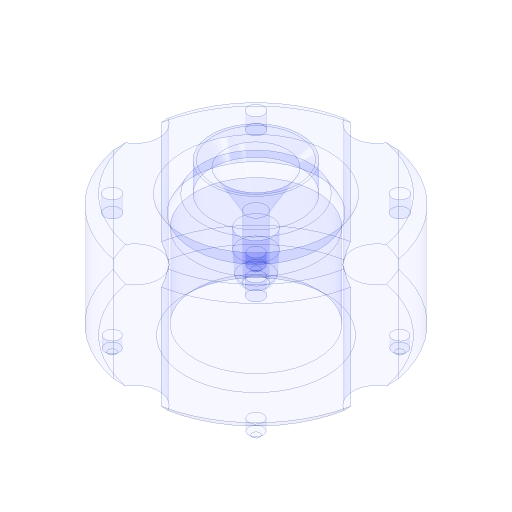
# Autodesk Inventor part: cpd_lowrcf_1.3_p3_20230620
Saved by Autodesk Inventor 2024 (Build 280153000, 153)
## iProperties
Created: 2021-12-08
Part Number: cpd_lowrcf_1.3_p3_20230620
Material: Generic
Document SubType Name: Modeling
Designer: tomos
Density: 1 g/cm^3
Appearance: Clear - Blue
Author: tomos
Autodesk Inventor part; units mm, degrees
ref_plane "YZ Plane" through (0, 0, 0) normal (1, 0, 0) x (0, 1, 0)
ref_plane "XZ Plane" through (0, 0, 0) normal (0, 1, 0) x (-1, 0, 0)
sketch "Sketch1" plane through (0, 0, 0) normal (0, 0, 1) x (1, 0, 0)
  line L0 (0, 0) -> (0, 22.2922) construction
  line L1 (0, 0) -> (22.0718, 0) construction
  line L2 (1, 4.659) -> (1, 11.1557)
  line L3 (1, 11.1557) -> (3.6, 15.659)
  line L4 (3.6, 15.659) -> (4.6, 15.659)
  line L5 (4.6, 15.659) -> (4.6, 12.659)
  line L6 (4.6, 12.659) -> (5.5, 12.659)
  line L7 (5.5, 12.659) -> (6.5, 10.9269)
  line L8 (6.5, 10.9269) -> (7.5, 12.659)
  line L9 (7.5, 12.659) -> (12.5, 12.659)
  line L10 (12.5, 12.659) -> (12.5, 0)
  line L11 (8.5, 0) -> (8.5, 0)
  line L12 (8.5, 0) -> (6.275, 0)
  line L13 (6.275, 0) -> (6.275, 9.659)
  line L14 (6.275, 9.659) -> (1.725, 9.659)
  line L15 (1.535, 4.659) -> (1, 4.659)
  line L16 (8.5, 0) -> (12.5, 0)
  line L17 (1.725, 9.659) -> (1.725, 7.659)
  line L18 (1.725, 7.659) -> (1.535, 4.659)
  dimension "d0" = 12.5
  dimension "d1" = 8.5
  dimension "d4" = 1
  dimension "d5" = 5
  dimension "d6" = 6.275
  dimension "d7" = 30
  dimension "d8" = 3
  dimension "d9" = 4.6
  dimension "d10" = 1
  dimension "d12" = 0
  dimension "d13" = 12.659
  dimension "d14" = 6.5
  dimension "d15" = 60
  dimension "d16" = 2
  dimension "d51" = 1.725
  dimension "d52" = 1.535
  dimension "d53" = 2
  dimension "d54" = 3
  constraints: 38 end point, 5 perpendicular, 4 point on line, 4 vertical, 2 horizontal, 1 parallel
  measures "d0" distance between parallel lines of L10 L0
  measures "d1" distance between parallel lines of L11 L0
  measures "d4" distance between parallel lines of L2 L0
  measures "d5" distance between parallel lines of L15 L14
  measures "d6" distance between parallel lines of L13 L0
  measures "d7" angle of L3 L0
  measures "d8" distance of L4.end L5.end
  measures "d9" distance between parallel lines of L5 L0
  measures "d10" distance of L3.end L4.end
  measures "d12" distance between parallel lines of L16 L1
  measures "d13" distance between parallel lines of L16 L9
  measures "d14" distance from line of L7.end L0
  measures "d15" angle of L8 L7
  measures "d16" distance of L8.end L6.end
  measures "d51" distance between parallel lines of L0 L17
  measures "d52" distance from line of L0 L15.start
  measures "d53" distance of L14.end L17.end
  measures "d54" distance between parallel lines of L14 L9
revolve "Revolution1" add sketch "Sketch1" angle 360 about axis through (0, 0, 0) along (0, 1, 0)
chamfer "Chamfer1" distance 0.75 angle 45 1 edges at (-3.6, 15.659, 0)
fillet "Fillet1" radius 1 1 edges at (-1.535, 4.659, 0)
chamfer "Chamfer2" distance 1 angle 45 3 edges at (-12.5, 12.659, 0) (-12.5, 0, 0) (-6.275, 0, 0)
sketch "Sketch4" plane through (0, 0, 0) normal (0, -1, 0) x (1, 0, 0)
  circle A0 centre (0, 0) radius 1 construction
  circle A1 centre (0, 0) radius 10.5 construction
  circle A2 centre (0, 0) radius 12.5 construction
  line L0 (0, 14.7546) -> (0, 0) construction
  line L1 (0, 0) -> (12.5, 12.5) construction
  circle A3 centre (7.4246, 7.4246) radius 0.75
  dimension "d55" = 21
  dimension "d56" = 45
  dimension "d57" = 1.5
  constraints: 4 end point, 2 coincident, 1 centre point, 1 point on line, 1 vertical, 3 other
  measures "d56" angle of L0 L1
  measures "d57" diameter of A3
extrude "Extrusion4" add sketch "Sketch4" along normal blind 1.5
chamfer "Chamfer5" distance 0.35 angle 45 1 edges at (6.6746, -1.5, 7.4246)
pattern_circular "Circular Pattern3" count 4 over 360 about axis through (0, 13.4073, 0) along (0, -1, 0) of "Extrusion4", "Chamfer5"
sketch "Sketch5" plane through (0, 0, 0) normal (0, -1, 0) x (1, 0, 0)
  circle A0 centre (0, 0) radius 10.5 construction
  line L0 (0, 0) -> (0, 19.578) construction
  line L1 (0, 0) -> (13.2063, 13.2063) construction
  circle A1 centre (0, 0) radius 1 construction
  line L2 (0, 0) -> (-14.8973, 0) construction
  circle A2 centre (0, 0) radius 12.5 projected
  circle A3 centre (0, 12.5) radius 2.5
  point P0 (7.4246, 7.4246)
  point P1 (-2.4875, 12.25)
  point P2 (2.4875, 12.25)
  dimension "d66" = 21
  dimension "d67" = 45
  dimension "d68" = 5
  constraints: 6 end point, 2 point on line, 1 centre point, 1 coincident, 1 horizontal, 1 vertical, 5 other
  measures "d67" angle of L0 L1
  measures "d68" diameter of A3
extrude "Extrusion5" cut sketch "Sketch5" against normal blind 12.659 contours A3 A2 picked at (0, 11.6481)
pattern_circular "Circular Pattern4" count 4 over 360 about axis through (0, 13.4073, 0) along (0, -1, 0) of "Extrusion5"
sketch "Sketch6" plane through (0, 12.659, 12.5) normal (0, 1, 0) x (1, 0, 0)
  circle A0 centre (0, 12.5) radius 1 construction
  circle A1 centre (0, 12.5) radius 10.5 construction
  line L0 (0, 12.5) -> (0, 36.8788) construction
  line L1 (0, 12.5) -> (13.3932, 25.8932) construction
  circle A2 centre (7.4246, 19.9246) radius 0.8
  dimension "d74" = 21
  dimension "d75" = 45
  dimension "d76" = 1.6
  constraints: 4 end point, 2 coincident, 1 centre point, 1 point on line, 1 vertical, 3 other
  measures "d75" angle of L0 L1
  measures "d76" diameter of A2
extrude "Extrusion6" cut sketch "Sketch6" against normal blind 1.7
pattern_circular "Circular Pattern5" count 4 over 360 about axis through (0, 7.9073, 0) along (0, -1, 0) of "Extrusion6"
ref_plane "Work Plane2" through (-2.4875, 0, 12.25) normal (-0.1989975, 0, 0.98) x (0, -1, 0)
sketch "Sketch9" plane through (-2.4875, 0, 12.25) normal (-0.1989975, 0, 0.98) x (0, -1, 0)
  line L0 (-8.6342, 3.9668) -> (-3.8448, 3.9668) construction
  line L1 (-3.8448, 3.9668) -> (-3.8448, 0.9089) construction
  line L2 (-3.8448, 0.9089) -> (-8.6342, 0.9089) construction
  line L3 (-8.6342, 0.9089) -> (-8.6342, 3.9668) construction
  point P0 (0, 0)
  dimension "d25" = 45
  dimension "d27" = 5
  dimension "d29" = 1.5
  constraints: 4 end point, 2 centre point, 2 coincident, 2 point on line, 1 horizontal, 6 other
  measures "d25" angle of L0 L1
sketch "Sketch3" plane through (-12.5, 12.659, 0) normal (0, 1, 0) x (1, 0, 0)
  circle A0 centre (12.5, 0) radius 1 construction
  circle A1 centre (12.5, 0) radius 10.5 construction
  line L0 (12.5, 0) -> (30.51, 0) construction
  line L1 (12.5, 0) -> (26.5897, -14.0897) construction
  circle A2 centre (19.9246, -7.4246) radius 0.8
  dimension "d40" = 45
  dimension "d41" = 21
  dimension "d42" = 1.6
  constraints: 4 end point, 2 centre point, 2 coincident, 1 horizontal
  measures "d40" angle of L1 L0
  measures "d41" diameter of A1
  measures "d42" diameter of A2
equation "\"cutpipette_length\" = 5.7"
body "Solid1"
